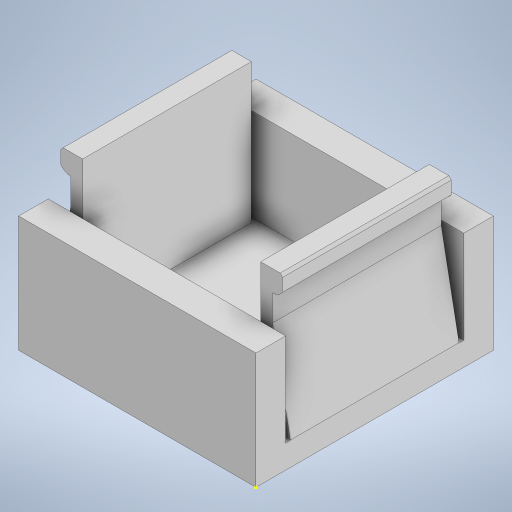
# Autodesk Inventor part: boxtest2
Saved by Autodesk Inventor 2023 (Build 270158000, 158)
## iProperties
Created: 2022-12-05
Part Number: boxtest2
Material: Generic
Document SubType Name: Modeling
Designer: spfow
Density: 1 g/cm^3
Appearance: Default
Author: spfow
Autodesk Inventor part; units mm, degrees
ref_plane "YZ Plane" through (0, 0, 0) normal (1, 0, 0) x (0, 1, 0)
ref_plane "XZ Plane" through (0, 0, 0) normal (0, 1, 0) x (-1, 0, 0)
ref_plane "XY Plane" through (0, 0, 0) normal (0, 0, 1) x (1, 0, 0)
sketch "Sketch1" plane through (0, 0, 0) normal (0, 1, 0) x (-1, 0, 0)
  point P0 (0, 0)
sketch "Sketch2" plane through (0, 0, 0) normal (0, 1, 0) x (-1, 0, 0)
  line L0 (0, 0) -> (25.4, 0)
  line L1 (25.4, 0) -> (25.4, -25.4)
  line L2 (25.4, -25.4) -> (0, -25.4)
  line L3 (0, -25.4) -> (0, 0)
  dimension "d0" = 25.4
  dimension "d1" = 25.4
  constraints: 8 end point, 2 parallel, 1 horizontal, 1 perpendicular
  measures "d0" distance of L1.end L2.end
  measures "d1" distance of L0.end L1.end
extrude "Extrusion1" add sketch "Sketch2" along normal blind 17.78
sketch "Sketch3" plane through (0, 17.78, 0) normal (0, 1, 0) x (1, 0, 0)
  line L0 (-22.225, 3.175) -> (-3.175, 3.175)
  line L1 (-3.175, 3.175) -> (-3.175, 22.225)
  line L2 (-3.175, 22.225) -> (-22.225, 22.225)
  line L3 (-22.225, 22.225) -> (-22.225, 3.175)
  line L4 (-25.4, 25.4) -> (-25.4, 0) projected
  line L5 (0, 25.4) -> (-25.4, 25.4) projected
  line L6 (-25.4, 0) -> (0, 0) projected
  line L7 (0, 0) -> (0, 25.4) projected
  dimension "d4" = 3.175
  dimension "d5" = 3.175
  dimension "d6" = 3.175
  dimension "d7" = 3.175
  constraints: 8 end point, 2 parallel, 1 horizontal, 1 perpendicular
  measures "d4" distance between parallel lines of L4 L3
  measures "d5" distance between parallel lines of L5 L2
  measures "d6" distance between parallel lines of L6 L0
  measures "d7" distance between parallel lines of L7 L1
extrude "Extrusion2" cut sketch "Sketch3" against normal blind 15.24 contours L3 L2 L1 L0
sketch "Sketch4" plane through (-25.4, 0, 0) normal (0, 0, 1) x (1, 0, 0)
  circle A0 centre (1.905, 16.51) radius 1.27
  circle A1 centre (23.495, 16.51) radius 1.27
  line L0 (0, 17.78) -> (25.4, 17.78) projected
  line L1 (3.175, 17.78) -> (3.175, 2.54) projected
  line L2 (22.225, 17.78) -> (22.225, 2.54) projected
  line L3 (3.175, 17.78) -> (1.905, 17.78)
  line L4 (1.905, 17.78) -> (1.905, 12.446)
  line L5 (1.905, 12.446) -> (3.175, 12.446)
  line L6 (3.175, 12.446) -> (3.175, 17.78)
  line L7 (22.225, 17.78) -> (23.495, 17.78)
  line L8 (23.495, 17.78) -> (23.495, 12.446)
  line L9 (23.495, 12.446) -> (22.225, 12.446)
  line L10 (22.225, 12.446) -> (22.225, 17.78)
  line L11 (3.175, 17.78) -> (0, 17.78)
  line L12 (0, 17.78) -> (0, 12.446)
  line L13 (0, 12.446) -> (3.175, 12.446)
  line L14 (3.175, 12.446) -> (3.175, 17.78)
  line L15 (22.225, 17.78) -> (25.4, 17.78)
  line L16 (25.4, 17.78) -> (25.4, 12.446)
  line L17 (25.4, 12.446) -> (22.225, 12.446)
  line L18 (22.225, 12.446) -> (22.225, 17.78)
  point P0 (25.4, 0)
  point P1 (1.905, 12.446)
  point P2 (1.905, 15.24)
  point P3 (1.905, 17.78)
  point P4 (23.495, 15.24)
  dimension "d10" = 2.54
  dimension "d11" = 2.54
  dimension "d12" = 1.27
  dimension "d13" = 1.27
  dimension "d14" = 1.27
  dimension "d15" = 1.27
  dimension "d16" = 1.27
  dimension "d17" = 5.334
  dimension "d18" = 1.27
  dimension "d19" = 5.334
  constraints: 32 end point, 8 parallel, 4 horizontal, 4 perpendicular, 2 centre point, 1 point on line
  measures "d10" diameter of A0
  measures "d11" diameter of A1
  measures "d12" distance from line of L0 A1.centre
  measures "d13" distance from line of L0 A0.centre
  measures "d14" distance from line of L1 A0.centre
  measures "d15" distance from line of L2 A1.centre
  measures "d16" distance of L5.end L4.end
  measures "d17" distance of L3.end L4.end
  measures "d18" distance of L8.end L9.end
  measures "d19" distance of L7.end L8.end
extrude "Extrusion3" cut sketch "Sketch4" against normal blind 25.4 contours A0 L4 L13 L12 L0 | L0 L16 L17 L8 A1
sketch "Sketch5" plane through (0, 0, 0) normal (1, 0, 0) x (0, 0, -1)
  line L0 (3.175, 17.78) -> (22.225, 17.78) projected
  line L1 (0, 12.446) -> (25.4, 12.446) projected
  line L2 (0, 12.446) -> (25.4, 12.446) projected
  line L3 (0, 17.78) -> (3.675, 17.78)
  line L4 (3.675, 17.78) -> (3.675, 12.446)
  line L5 (3.675, 12.446) -> (0, 12.446)
  line L6 (0, 12.446) -> (0, 17.78)
  line L7 (25.4, 15.24) -> (25.4, 17.78) projected
  line L8 (25.4, 17.78) -> (21.725, 17.78)
  line L9 (21.725, 17.78) -> (21.725, 12.446)
  line L10 (21.725, 12.446) -> (25.4, 12.446)
  line L11 (25.4, 12.446) -> (25.4, 17.78)
  line L12 (22.225, 2.54) -> (3.175, 2.54) projected
  line L13 (3.675, 12.446) -> (3.175, 12.446)
  line L14 (3.175, 12.446) -> (3.175, 2.54)
  line L15 (3.175, 2.54) -> (3.675, 2.54)
  line L16 (3.675, 2.54) -> (3.675, 12.446)
  line L17 (22.225, 17.78) -> (22.225, 2.54) projected
  line L18 (21.725, 12.446) -> (22.225, 12.446)
  line L19 (22.225, 12.446) -> (22.225, 2.54)
  line L20 (22.225, 2.54) -> (21.725, 2.54)
  line L21 (21.725, 2.54) -> (21.725, 12.446)
  point P0 (0, 0)
  point P1 (25.4, 12.446)
  point P2 (21.725, 12.446)
  point P3 (0, 12.446)
  point P4 (22.225, 12.446)
  dimension "d25" = 3.675
  dimension "d26" = 3.675
  constraints: 32 end point, 8 parallel, 4 horizontal, 4 perpendicular, 2 point on line
  measures "d25" distance of L4.end L5.end
  measures "d26" distance of L10.end L9.end
extrude "Extrusion4" cut sketch "Sketch5" against normal blind 25.4 contours L0 L4 L1 L6 L3 | L0 L17 L1 L9 | L16 L12 L14 L1 | L8 L7 L11 L1 L17 | L1 L17 L12 L21
sketch "Sketch7" plane through (0, 2.54, -3.675) normal (0, 0, 1) x (1, 0, 0)
  line L0 (-3.175, 15.24) -> (-3.175, 0) projected
  line L1 (-1.905, 12.7) -> (-1.905, 9.906) projected
  line L2 (0, 9.906) -> (0, 0) projected
  line L3 (-1.905, 9.906) -> (0, 9.906) projected
  line L4 (0, 0) -> (-1.905, 9.906)
  line L5 (-1.905, 9.906) -> (0, 9.906)
  line L6 (0, 0) -> (-25.4, 0) projected
  line L7 (0, 0) -> (0, 9.906)
  line L8 (0, 9.906) -> (-25.4, 9.906) projected
  line L9 (-25.4, 9.906) -> (-25.4, 0)
  line L10 (-23.495, 9.906) -> (-23.495, 12.7) projected
  line L11 (-25.4, 0) -> (-23.495, 9.906)
  line L12 (-23.495, 9.906) -> (-25.4, 9.906)
  point P0 (0, -2.54)
  constraints: 12 end point, 3 perpendicular, 1 collinear
extrude "Extrusion6" cut sketch "Sketch7" against normal blind 18.5 contours L3 L2 L4 | L11 L9 L8
sketch "Sketch8" plane through (-23.495, 17.78, -3.675) normal (0, 0, 1) x (1, 0, 0)
  arc A0 (0, 0) -> (0, -2.54) centre (0, -1.27) ccw projected
  line L0 (-1.07, -2.27) -> (-1.07, 0)
  line L1 (-1.07, 0) -> (-1.27, 0)
  line L2 (-1.27, 0) -> (-1.27, -1.27)
  line L3 (-1.07, 0) -> (-1.07, -2.27)
  line L4 (-1.07, -2.27) -> (-1.27, -2.27)
  line L5 (-1.27, -2.27) -> (-1.27, -1.27)
  arc A1 (21.59, -2.54) -> (21.59, 0) centre (21.59, -1.27) ccw projected
  line L6 (22.66, -1.3632) -> (22.66, 0)
  line L7 (22.66, 0) -> (22.86, 0)
  line L8 (22.86, 0) -> (22.86, -1.27)
  line L9 (22.86, -1.3632) -> (22.86, -3.2076)
  line L10 (22.86, -3.2076) -> (22.66, -3.2076)
  line L11 (22.66, -3.2076) -> (22.66, -1.3632)
  line L12 (22.86, 0) -> (-1.27, 0)
  line L13 (-1.27, 0) -> (-1.27, -0.3)
  line L14 (-1.27, -0.3) -> (22.86, -0.3)
  line L15 (22.86, -0.3) -> (22.86, 0)
  line L16 (0, 0) -> (1.27, 0) projected
  point P0 (23.495, -17.78)
  point P1 (10.795, -0.3)
  point P2 (22.66, -1.9541)
  point P3 (22.66, -0.5859)
  point P4 (-1.07, 0)
  point P5 (-1.07, -0.3)
  point P6 (22.86, -0.3)
  point P7 (22.66, 0)
  dimension "d34" = 0.2
  dimension "d35" = 1
  dimension "d36" = 0.2
  dimension "d37" = 0.3
  dimension "d38" = 0
  constraints: 32 end point, 6 parallel, 2 point on circle, 2 point on line, 1 horizontal, 1 midpoint, 1 perpendicular
  measures "d34" distance of L0.end L1.end
  measures "d35" distance of L4.end L2.end
  measures "d36" distance of L6.end L7.end
  measures "d37" distance from line of point (10.795, -0.3) L12
  measures "d38" distance between parallel lines of L16 L12
extrude "Extrusion7" cut sketch "Sketch8" against normal blind 18.5 contours L12 A1 L14 A0 | A0 L14 L0 L12 | L0 L14 L2 L1 | L0 A0 | A0 L2 L14 L0 | A1 L12 L6 L14 | A0 L0 L4 L5 | A1 L11 L6 | L6 L7 L8 L14
body "Solid1"
